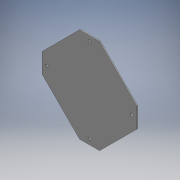
# Autodesk Inventor part: separatingPanels
Saved by Autodesk Inventor 2016 (Build 200138000, 138)
## iProperties
Created: 2016-07-21
Part Number: separatingPanels
Material: Generic
Document SubType Name: Modeling
Designer: Jonathan
Density: 1 g/cm^3
Appearance: Default
Author: Jonathan
Autodesk Inventor part; units mm, degrees
ref_plane "YZ Plane" through (0, 0, 0) normal (1, 0, 0) x (0, 1, 0)
ref_plane "XZ Plane" through (0, 0, 0) normal (0, 1, 0) x (-1, 0, 0)
ref_plane "XY Plane" through (0, 0, 0) normal (0, 0, 1) x (1, 0, 0)
sketch "Sketch1" plane through (0, 0, 0) normal (0, 1, 0) x (-1, 0, 0)
  line L0 (95, -95) -> (-95, -95)
  line L1 (-95, -95) -> (-95, 95)
  line L2 (-95, 95) -> (95, 95)
  line L3 (95, 95) -> (95, -95)
  line L4 (95, -95) -> (-95, 95) construction
  line L5 (-95, -95) -> (95, 95) construction
  point P0 (0, 0)
  point P1 (0, 0)
  point P2 (0, 0)
  dimension "d25" = 190
  constraints: 12 end point, 3 midpoint, 2 parallel, 2 perpendicular, 1 coincident, 1 horizontal
  measures "d25" distance of L0.end L1.end
extrude "Extrusion1" add sketch "Sketch1" along normal blind 1.5875
sketch "Sketch2" plane through (0, 1.5875, 0) normal (0, 1, 0) x (1, 0, 0)
  line L0 (-95, -95) -> (95, -95) projected
  point P0 (0, 0)
  point P1 (0, -85)
  dimension "d26" = 10
  constraints: 1 vertical alignment
  measures "d26" distance from line of L0 point (0, -85)
hole "Hole1" at (0, 1.5875, 85) direction (0, -1, 0) diameter 5.5 end through all clearance for "Socket Head Cap Screw" size "M5" standard "Ansi Metric M Profile"
mirror "Mirror1" about plane through (0, 0, 0) normal (1, 0, 0) of "Hole1"
pattern_circular "Circular Pattern1" count 4 over 360 about axis through (0, -10, 0) along (0, 1, 0) of "Hole1", "Mirror1"
chamfer "Chamfer1" distance 75 angle 45 4 edges at (95, 0.7937, -95) (95, 0.7937, 95) (-95, 0.7937, 95) (-95, 0.7937, -95)
equation "\"d22\" = panelChamfer"
equation "\"panelChamfer\" = 75"
body "Solid1"
